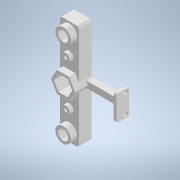
# Autodesk Inventor part: priključek za matice
Saved by Autodesk Inventor 2022 (Build 260153000, 153)
## iProperties
Created: 2022-03-05
Part Number: priključek za matice
Material: Generic
Document SubType Name: Modeling
Designer: simon
Density: 1 g/cm^3
Appearance: Default
Author: simon
Autodesk Inventor part; units mm, degrees
ref_plane "YZ Plane" through (0, 0, 0) normal (1, 0, 0) x (0, 1, 0)
ref_plane "XZ Plane" through (0, 0, 0) normal (0, 1, 0) x (-1, 0, 0)
ref_plane "XY Plane" through (0, 0, 0) normal (0, 0, 1) x (1, 0, 0)
sketch "Sketch1" plane through (0, 0, 0) normal (0, 0, 1) x (1, 0, 0)
  arc A0 (-5.5, 41.2) -> (-7.5, 39.2) centre (-5.5, 39.2) ccw
  line L0 (-7.5, 39.2) -> (-7.5, -39.2)
  arc A1 (-7.5, -39.2) -> (-5.5, -41.2) centre (-5.5, -39.2) ccw
  line L1 (-5.5, -41.2) -> (5.5, -41.2)
  arc A2 (5.5, -41.2) -> (7.5, -39.2) centre (5.5, -39.2) ccw
  line L2 (7.5, -39.2) -> (7.5, 39.2)
  arc A3 (7.5, 39.2) -> (5.5, 41.2) centre (5.5, 39.2) ccw
  line L3 (5.5, 41.2) -> (-5.5, 41.2)
  circle A4 centre (0, 0) radius 5
  circle A5 centre (0, 0) radius 6.25
  line L4 (-3.6084, -6.25) -> (-7.2169, 0)
  line L5 (-7.2169, 0) -> (-3.6084, 6.25)
  line L6 (-3.6084, 6.25) -> (3.6084, 6.25)
  line L7 (3.6084, 6.25) -> (7.2169, 0)
  line L8 (7.2169, 0) -> (3.6084, -6.25)
  line L9 (3.6084, -6.25) -> (-3.6084, -6.25)
  line L10 (-8, 40) -> (-8, -40)
  line L11 (-8, -40) -> (8, -40)
  line L12 (8, -40) -> (8, 40)
  line L13 (8, 40) -> (-8, 40)
  line L14 (-8, 40) -> (8, -40) construction
  line L15 (-8, -40) -> (8, 40) construction
  circle A6 centre (0, 33.7) radius 4.05
  arc A7 (-3.7293, -35.1464) -> (3.6861, -35.2533) centre (0, -33.7) ccw
  arc A8 (3.7293, -32.2536) -> (-3.6861, -32.1467) centre (0, -33.7) ccw
  arc A9 (3.6861, -35.2533) -> (3.7293, -32.2536) centre (0, -33.7) ccw
  arc A10 (-3.6861, -32.1467) -> (-3.7293, -35.1464) centre (0, -33.7) ccw
  line L16 (4.7631, -8.25) -> (9.5263, 0)
  line L17 (9.5263, 0) -> (4.7631, 8.25)
  line L18 (4.7631, 8.25) -> (-4.7631, 8.25)
  line L19 (-4.7631, 8.25) -> (-9.5263, 0)
  line L20 (-9.5263, 0) -> (-4.7631, -8.25)
  line L21 (-4.7631, -8.25) -> (4.7631, -8.25)
  arc A11 (-20.5703, 32.4401) -> (-22.678, 30.5539) centre (-20.681, 30.4432) ccw
  line L22 (-9.7869, 31.8423) -> (-20.5703, 32.4401)
  arc A12 (-9.7869, 31.8423) -> (-7.6792, 33.7285) centre (-9.6762, 33.8392) ccw
  line L23 (-7.3471, 39.7193) -> (-7.6792, 33.7285)
  arc A13 (-5.2395, 41.6055) -> (-7.3471, 39.7193) centre (-5.3502, 39.6086) ccw
  line L24 (13.5317, 40.5648) -> (-5.2395, 41.6055)
  arc A14 (15.4179, 38.4572) -> (13.5317, 40.5648) centre (13.421, 38.5679) ccw
  line L25 (15.0858, 32.4664) -> (15.4179, 38.4572)
  arc A15 (15.0858, 32.4664) -> (16.972, 30.3587) centre (17.0827, 32.3557) ccw
  line L26 (27.7555, 29.7609) -> (16.972, 30.3587)
  arc A16 (29.6417, 27.6532) -> (27.7555, 29.7609) centre (27.6448, 27.764) ccw
  line L27 (28.4128, 5.4873) -> (29.6417, 27.6532)
  arc A17 (28.4128, 5.4873) -> (30.299, 3.3796) centre (30.4097, 5.3766) ccw
  line L28 (116.1672, -1.3809) -> (30.299, 3.3796)
  arc A18 (116.1672, -1.3809) -> (118.2748, 0.5053) centre (116.2779, 0.616) ccw
  line L29 (119.5037, 22.6713) -> (118.2748, 0.5053)
  arc A19 (121.6113, 24.5575) -> (119.5037, 22.6713) centre (121.5006, 22.5605) ccw
  line L30 (133.7926, 23.8821) -> (121.6113, 24.5575)
  arc A20 (135.6789, 21.7745) -> (133.7926, 23.8821) centre (133.6819, 21.8852) ccw
  line L31 (135.3467, 15.7837) -> (135.6789, 21.7745)
  arc A21 (135.3467, 15.7837) -> (137.2329, 13.676) centre (137.3437, 15.673) ccw
  line L32 (153.2084, 12.7904) -> (137.2329, 13.676)
  arc A22 (153.2084, 12.7904) -> (155.3161, 14.6766) centre (153.3191, 14.7873) ccw
  line L33 (155.6482, 20.6674) -> (155.3161, 14.6766)
  arc A23 (157.7558, 22.5536) -> (155.6482, 20.6674) centre (157.6451, 20.5567) ccw
  line L34 (169.9371, 21.8783) -> (157.7558, 22.5536)
  arc A24 (171.8233, 19.7706) -> (169.9371, 21.8783) centre (169.8264, 19.8813) ccw
  line L35 (171.2144, 8.7875) -> (171.8233, 19.7706)
  arc A25 (169.1068, 6.9013) -> (171.2144, 8.7875) centre (169.2175, 8.8982) ccw
  line L36 (168.1083, 6.9566) -> (169.1068, 6.9013)
  arc A26 (168.1083, 6.9566) -> (166.0007, 5.0704) centre (167.9976, 4.9597) ccw
  line L37 (164.4286, -23.2861) -> (166.0007, 5.0704)
  arc A27 (164.4286, -23.2861) -> (166.3148, -25.3937) centre (166.4255, -23.3968) ccw
  line L38 (167.3133, -25.4491) -> (166.3148, -25.3937)
  arc A28 (169.1995, -27.5567) -> (167.3133, -25.4491) centre (167.2026, -27.446) ccw
  line L39 (168.5906, -38.5398) -> (169.1995, -27.5567)
  arc A29 (166.4829, -40.4261) -> (168.5906, -38.5398) centre (166.5937, -38.4291) ccw
  line L40 (154.3016, -39.7507) -> (166.4829, -40.4261)
  arc A30 (152.4154, -37.6431) -> (154.3016, -39.7507) centre (154.4124, -37.7538) ccw
  line L41 (152.8583, -29.6553) -> (152.4154, -37.6431)
  line L42 (132.8889, -28.5482) -> (152.8583, -29.6553)
  line L43 (132.4461, -36.536) -> (132.8889, -28.5482)
  arc A31 (130.3384, -38.4222) -> (132.4461, -36.536) centre (130.4492, -36.4253) ccw
  line L44 (118.1572, -37.7468) -> (130.3384, -38.4222)
  arc A32 (116.2709, -35.6392) -> (118.1572, -37.7468) centre (118.2679, -35.7499) ccw
  line L45 (117.4998, -13.4732) -> (116.2709, -35.6392)
  arc A33 (117.4998, -13.4732) -> (115.6136, -11.3656) centre (115.5029, -13.3625) ccw
  line L46 (29.7455, -6.605) -> (115.6136, -11.3656)
  arc A34 (29.7455, -6.605) -> (27.6378, -8.4913) centre (29.6348, -8.602) ccw
  line L47 (26.4089, -30.6572) -> (27.6378, -8.4913)
  arc A35 (24.3013, -32.5434) -> (26.4089, -30.6572) centre (24.412, -30.5465) ccw
  line L48 (13.5178, -31.9456) -> (24.3013, -32.5434)
  arc A36 (13.5178, -31.9456) -> (11.4102, -33.8318) centre (13.4071, -33.9425) ccw
  line L49 (11.0781, -39.8226) -> (11.4102, -33.8318)
  arc A37 (8.9704, -41.7088) -> (11.0781, -39.8226) centre (9.0811, -39.7119) ccw
  line L50 (-9.8008, -40.6682) -> (8.9704, -41.7088)
  arc A38 (-11.687, -38.5605) -> (-9.8008, -40.6682) centre (-9.69, -38.6712) ccw
  line L51 (-11.3548, -32.5697) -> (-11.687, -38.5605)
  arc A39 (-11.3548, -32.5697) -> (-13.2411, -30.4621) centre (-13.3518, -32.459) ccw
  line L52 (-24.0245, -29.8642) -> (-13.2411, -30.4621)
  arc A40 (-25.9107, -27.7566) -> (-24.0245, -29.8642) centre (-23.9138, -27.8673) ccw
  line L53 (-24.9586, -10.583) -> (-25.9107, -27.7566)
  arc A41 (-22.851, -8.6967) -> (-24.9586, -10.583) centre (-22.9617, -10.6937) ccw
  line L54 (-19.8556, -8.8628) -> (-22.851, -8.6967)
  line L55 (-18.7485, 11.1065) -> (-19.8556, -8.8628)
  line L56 (-21.7439, 11.2726) -> (-18.7485, 11.1065)
  arc A42 (-23.6301, 13.3802) -> (-21.7439, 11.2726) centre (-21.6331, 13.2695) ccw
  line L57 (-22.678, 30.5539) -> (-23.6301, 13.3802)
  circle A43 centre (0, 0) radius 5
  point P0 (0, 0)
  point P1 (0, -6.25)
  point P2 (-7.5, -3.5096)
  point P3 (7.5, -3.5096)
  point P4 (7.5, 3.5096)
  point P5 (-7.5, 3.5096)
extrude "Extrusion1" add sketch "Sketch1" along normal blind 10 contours L3 L24 A3 L13 A13 A0 | A13 L13 A0 | L3 A3 L24 | L13 A13 L23 L0 A0 | L13 A3 L2 L17 L18 L19 L0 L23 A13 | L19 L18 L17 L2 L16 L21 L20 L0 | L0 L20 L10 L19 | L10 L20 L19 | L17 L12 L16 L2 | L17 L16 L12 | L20 L21 L16 L2 A2 L11 A1 L0 | L11 A2 L1 L50 A1 | L50 L1 A1
sketch "Sketch2" plane through (0, 0, 10) normal (0, 0, 1) x (1, 0, 0)
  arc A0 (-7.5, -39.2) -> (-5.5, -41.2) centre (-5.5, -39.2) ccw projected
  line L0 (-5.5, -41.2) -> (5.5, -41.2) projected
  arc A1 (5.5, -41.2) -> (7.5, -39.2) centre (5.5, -39.2) ccw projected
  line L1 (7.5, -39.2) -> (7.5, -3.5096) projected
  line L2 (7.5, -3.5096) -> (9.5263, 0) projected
  line L3 (9.5263, 0) -> (7.5, 3.5096) projected
  line L4 (7.5, 3.5096) -> (7.5, 39.2) projected
  arc A2 (7.5, 39.2) -> (5.5, 41.2) centre (5.5, 39.2) ccw projected
  line L5 (5.5, 41.2) -> (-5.5, 41.2) projected
  arc A3 (-5.5, 41.2) -> (-7.5, 39.2) centre (-5.5, 39.2) ccw projected
  line L6 (-7.5, 39.2) -> (-7.5, 3.5096) projected
  line L7 (-7.5, 3.5096) -> (-9.5263, 0) projected
  line L8 (-9.5263, 0) -> (-7.5, -3.5096) projected
  line L9 (-7.5, -3.5096) -> (-7.5, -39.2) projected
  circle A4 centre (0, 33.7) radius 4.05 projected
  circle A5 centre (0, -33.7) radius 4 projected
  line L10 (3.6084, -6.25) -> (-3.6084, -6.25) projected
  line L11 (-3.6084, -6.25) -> (-7.2169, 0) projected
  line L12 (-7.2169, 0) -> (-3.6084, 6.25) projected
  line L13 (-3.6084, 6.25) -> (3.6084, 6.25) projected
  line L14 (3.6084, 6.25) -> (7.2169, 0) projected
  line L15 (7.2169, 0) -> (3.6084, -6.25) projected
  line L16 (-9.5263, 0) -> (-7.5, -3.5096) projected
  line L17 (-7.5, 3.5096) -> (-9.5263, 0) projected
  line L18 (-4.7631, 8.25) -> (-9.5263, 0)
  line L19 (-9.5263, 0) -> (-4.7631, -8.25)
  line L20 (-4.7631, -8.25) -> (4.7631, -8.25)
  line L21 (4.7631, -8.25) -> (9.5263, 0)
  line L22 (9.5263, 0) -> (4.7631, 8.25)
  line L23 (4.7631, 8.25) -> (-4.7631, 8.25)
  circle A6 centre (0, 33.7) radius 6.05
  circle A7 centre (0, -33.7) radius 6
  line L24 (0, 27.65) -> (0, 8.25)
  circle A8 centre (0, 17.95) radius 1.25
  circle A9 centre (0, 17.95) radius 3.25
  line L25 (7.2169, 0) -> (3.6084, -6.25) projected
  line L26 (7.2169, 0) -> (-7.2169, 0)
  circle A10 centre (0, -17.95) radius 1.25
  circle A11 centre (0, -17.95) radius 3.25
  point P0 (0, 0)
  dimension "d11" = 2
  dimension "d12" = 2
  dimension "d13" = 2.5
  dimension "d14" = 2
  constraints: 16 end point, 5 centre point, 2 midpoint, 1 horizontal, 1 symmetric about line, 1 vertical alignment, 9 other
  measures "d12" radial gap between concentric circles of A5 A7
  measures "d13" diameter of A8
  measures "d14" radial gap between concentric circles of A8 A9
extrude "Extrusion2" add sketch "Sketch2" along normal blind 5 contours L8 L7 L18 L23 L22 L3 L2 L21 L20 L19 | A6 | A7
extrude "Extrusion4" add sketch "Sketch2" along normal blind 3 contours A9 L24 A8 | L24 A8 A9 | A11
sketch "Sketch5" plane through (0, 0, 0) normal (0, 0, -1) x (-1, 0, 0)
  arc A0 (7.5, 39.2) -> (5.5, 41.2) centre (5.5, 39.2) ccw projected
  line L0 (7.5, 39.2) -> (7.5, -39.2) projected
  arc A1 (5.5, -41.2) -> (7.5, -39.2) centre (5.5, -39.2) ccw projected
  line L1 (5.5, -41.2) -> (-5.5, -41.2) projected
  arc A2 (-7.5, -39.2) -> (-5.5, -41.2) centre (-5.5, -39.2) ccw projected
  line L2 (-7.5, -39.2) -> (-7.5, 39.2) projected
  arc A3 (-5.5, 41.2) -> (-7.5, 39.2) centre (-5.5, 39.2) ccw projected
  line L3 (-5.5, 41.2) -> (5.5, 41.2) projected
  circle A4 centre (0, 0) radius 5 projected
  line L4 (3.6084, -6.25) -> (7.2169, 0) projected
  line L5 (-3.6084, -6.25) -> (3.6084, -6.25) projected
  line L6 (7.2169, 0) -> (3.6084, 6.25) projected
  line L7 (3.6084, 6.25) -> (-3.6084, 6.25) projected
  arc A5 (7.5, 39.2) -> (5.5, 41.2) centre (5.5, 39.2) ccw projected
  line L8 (7.5, 39.2) -> (7.5, -39.2) projected
  arc A6 (5.5, -41.2) -> (7.5, -39.2) centre (5.5, -39.2) ccw projected
  line L9 (5.5, -41.2) -> (-5.5, -41.2) projected
  arc A7 (-7.5, -39.2) -> (-5.5, -41.2) centre (-5.5, -39.2) ccw projected
  line L10 (-7.5, -39.2) -> (-7.5, 39.2) projected
  arc A8 (-5.5, 41.2) -> (-7.5, 39.2) centre (-5.5, 39.2) ccw projected
  line L11 (-5.5, 41.2) -> (5.5, 41.2) projected
  circle A9 centre (0, 0) radius 5 projected
  line L12 (7.2169, 0) -> (3.6084, -6.25)
  line L13 (3.6084, -6.25) -> (-3.6084, -6.25)
  line L14 (-3.6084, -6.25) -> (-7.2169, 0)
  line L15 (-7.2169, 0) -> (-3.6084, 6.25)
  line L16 (-3.6084, 6.25) -> (3.6084, 6.25)
  line L17 (3.6084, 6.25) -> (7.2169, 0)
  point P0 (0, 0)
  point P1 (-3.6084, 6.25)
  constraints: 12 end point, 1 coincident, 13 other
extrude "Extrusion5" add sketch "Sketch5" against normal blind 2 contours L5 L14 L15 L7 L6 L4
sketch "Sketch6" plane through (7.5, 3.5096, 0) normal (1, 0, 0) x (0, 0, -1)
  line L0 (0, 0) -> (0, 35.6904) projected
  line L1 (0, 35.6904) -> (-10, 35.6904) projected
  line L2 (-10, 0) -> (-10, 35.6904) projected
  line L3 (0, 0) -> (-10, 0) projected
  line L4 (0, -42.7096) -> (0, -7.0192) projected
  line L5 (0, -7.0192) -> (-10, -7.0192) projected
  line L6 (-10, -42.7096) -> (-10, -7.0192) projected
  line L7 (0, -42.7096) -> (-10, -42.7096) projected
  line L8 (0, -3.5096) -> (0, 0) projected
  line L9 (0, 0) -> (-10, 0) projected
  line L10 (-10, 4.7404) -> (-10, 0) projected
  line L11 (-10, 4.7404) -> (-15, 4.7404) projected
  line L12 (-15, -3.5096) -> (-15, 4.7404) projected
  line L13 (0, -3.5096) -> (-15, -3.5096) projected
  line L14 (0, -7.0192) -> (0, -3.5096) projected
  line L15 (0, -3.5096) -> (-15, -3.5096) projected
  line L16 (-15, -11.7596) -> (-15, -3.5096) projected
  line L17 (-10, -11.7596) -> (-15, -11.7596) projected
  line L18 (-10, -7.0192) -> (-10, -11.7596) projected
  line L19 (0, -7.0192) -> (-10, -7.0192) projected
  line L20 (0, -3.5096) -> (-10, -3.5096)
  line L21 (0, -3.5096) -> (-15, -3.5096) projected
  line L22 (-10, -6.0096) -> (0, -6.0096)
  line L23 (0, -6.0096) -> (0, -1.0096)
  line L24 (0, -1.0096) -> (-10, -1.0096)
  line L25 (-10, -1.0096) -> (-10, -6.0096)
  line L26 (-10, -6.0096) -> (0, -1.0096) construction
  line L27 (0, -6.0096) -> (-10, -1.0096) construction
  line L28 (5, -13.5096) -> (5, 6.4904)
  line L29 (5, 6.4904) -> (-5, 6.4904)
  line L30 (-5, 6.4904) -> (-5, -13.5096)
  line L31 (-5, -13.5096) -> (5, -13.5096)
  line L32 (5, -13.5096) -> (-5, 6.4904) construction
  line L33 (5, 6.4904) -> (-5, -13.5096) construction
  line L34 (0, 0) -> (0, 35.6904) projected
  point P0 (-5, -3.5096)
  point P1 (-10, -16.0096)
  point P2 (0, -16.0096)
  point P3 (0, 8.9904)
  point P4 (-10, 8.9904)
  point P5 (-5, -1.0096)
  point P6 (-5, -6.0096)
  point P7 (0, 6.4904)
  point P8 (0, -13.5096)
  dimension "d19" = 5
  constraints: 26 end point, 6 parallel, 4 midpoint, 2 perpendicular, 2 point on line
  measures "d19" distance of L23.end L22.end
extrude "Extrusion6" add sketch "Sketch6" along normal blind 27.5 contours L8 L13 L30 L24 | L14 L22 L30 L13
sketch "Sketch12" plane through (0, 0, 10) normal (0, 0, 1) x (1, 0, 0)
  circle A0 centre (0, -17.95) radius 1.25 projected
  circle A1 centre (0, 17.95) radius 1.25 projected
  point P0 (0, 0)
extrude "Extrusion12" cut sketch "Sketch12" against normal blind 32.5
fillet "Fillet2" radius 2 2 edges at (8.0829, 2.5, 2.5) (8.0829, -2.5, 2.5)
sketch "Sketch21" plane through (35, 3.5096, 0) normal (1, 0, 0) x (0, 0, -1)
  line L0 (0, -1.0096) -> (-5, -1.0096) projected
  line L1 (-5, -1.0096) -> (-5, -6.0096) projected
  line L2 (-5, -6.0096) -> (0, -6.0096) projected
  line L3 (0, -6.0096) -> (0, -1.0096) projected
  line L4 (-5, -13.5096) -> (0, -13.5096)
  line L5 (0, -13.5096) -> (0, 6.4904)
  line L6 (0, 6.4904) -> (-5, 6.4904)
  line L7 (-5, 6.4904) -> (-5, -13.5096)
  line L8 (-5, -13.5096) -> (0, 6.4904) construction
  line L9 (0, -13.5096) -> (-5, 6.4904) construction
  line L10 (-5, -11.0096) -> (0, -11.0096)
  line L11 (0, -11.0096) -> (0, 3.9904)
  line L12 (0, 3.9904) -> (-5, 3.9904)
  line L13 (-5, 3.9904) -> (-5, -11.0096)
  line L14 (0, -3.5096) -> (-15, -3.5096) projected
  line L15 (-5, -11.0096) -> (0, 3.9904) construction
  line L16 (0, -11.0096) -> (-5, 3.9904) construction
  line L17 (-5, -1.0096) -> (0, -1.0096) projected
  circle A0 centre (-2.5, -11.0096) radius 1.5
  circle A1 centre (-2.5, 3.9904) radius 1.5
  line L18 (-5, 6.4904) -> (-10, 6.4904)
  line L19 (-10, 6.4904) -> (-10, -13.5096)
  line L20 (-10, -13.5096) -> (-5, -13.5096)
  line L21 (-5, -13.5096) -> (-5, 6.4904)
  point P0 (-2.5, -3.5096)
  point P1 (-2.5, -3.5096)
  point P2 (0, -6.0096)
  dimension "d84" = 20
  dimension "d85" = 15
  dimension "d86" = 3
  dimension "d87" = 3
  dimension "d88" = 5
  dimension "d89" = 5
  constraints: 32 end point, 7 midpoint, 7 parallel, 4 perpendicular, 2 centre point, 1 horizontal, 1 point on line
  measures "d84" distance of L5.end L4.end
  measures "d85" distance of L11.end L10.end
  measures "d86" diameter of A0
  measures "d87" diameter of A1
  measures "d88" distance between parallel lines of L5 L7
  measures "d89" distance of L20.end L19.end
extrude "Extrusion19" add sketch "Sketch21" along normal blind 2 contours L3 L14 L1 L0 | L0 L7 L12 A1 L5 | L1 L14 L19 L18 L7 | L3 L2 L1 L14 | L12 A1 L7 L6 L5 | L1 L7 L20 L19 L14 | L5 L10 A0 L7 L2 | L5 L4 L7 L10 A0
fillet "Fillet5" radius 2 6 edges at (36, -10, 10) (36, 10, 10) (36, -10, 0) (36, 10, 0) (35, 2.5, 2.5) (35, -2.5, 2.5)
body "Solid1"
